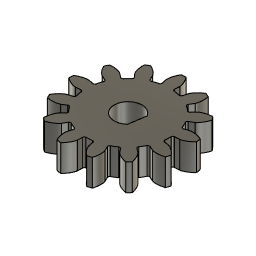
Spur Gear (13 teeth) (Autodesk Fusion 360 design; units mm, degrees)
description: Spur Gear; Module: 1.5; Num Teeth: 13; Pressure Angle: 20.0; Backlash: 0.15 mm
Autodesk Fusion 360 part; units mm, degrees
sketch "Sketch1" plane through (0, 0, 0) normal (0, 0, 1) x (1, 0, 0)
  circle A0 centre (0, 0) radius 7.8992
extrude "Extrude1" add sketch "Sketch1" along normal blind 5
sketch "Sketch2" plane through (0, 0, 0) normal (0, 0, 1) x (1, 0, 0)
  spline S0 degree 5 poles (9.0824, -1.2049) (9.0885, -1.2057) (9.1008, -1.2071) (9.1191, -1.2087) (9.1437, -1.2097) (9.1746, -1.2095) (9.2055, -1.2083) (9.2365, -1.2064) (9.2675, -1.2041) (9.2986, -1.2016) (9.3296, -1.1988) (9.3607, -1.1957) (9.3919, -1.1921) (9.423, -1.1881) (9.4542, -1.1835) (9.4854, -1.1784) (9.5166, -1.1729) (9.5478, -1.167) (9.5791, -1.1608) (9.6103, -1.1544) (9.6416, -1.1476) (9.6728, -1.1405) (9.7041, -1.1331) (9.7353, -1.1254) (9.7665, -1.1174) (9.7978, -1.109) (9.829, -1.1003) (9.8603, -1.0913) (9.8915, -1.0821) (9.9227, -1.0726) (9.9539, -1.0628) (9.9851, -1.0527) (10.0163, -1.0424) (10.0475, -1.0317) (10.0786, -1.0209) (10.1098, -1.0097) (10.1409, -0.9983) (10.172, -0.9866) (10.2031, -0.9747) (10.2342, -0.9626) (10.2652, -0.9501) (10.2962, -0.9375) (10.3272, -0.9246) (10.3582, -0.9114) (10.3892, -0.898) (10.4201, -0.8844) (10.451, -0.8706) (10.4819, -0.8565) (10.5127, -0.8421) (10.5435, -0.8276) (10.5743, -0.8128) (10.605, -0.7978) (10.6357, -0.7825) (10.6664, -0.7671) (10.6971, -0.7514) (10.7277, -0.7355) (10.7582, -0.7193) (10.7888, -0.703) (10.8193, -0.6864) (10.8497, -0.6696) (10.8801, -0.6526) (10.9105, -0.6354) (10.9409, -0.618) (10.9711, -0.6004) (11.0014, -0.5825) (11.0316, -0.5645) (11.0618, -0.5462) (11.0919, -0.5277) (11.1219, -0.5091) (11.1519, -0.4902) (11.1819, -0.4711) (11.2058, -0.4557) (11.2238, -0.444) (11.2357, -0.4362) (11.2417, -0.4323) knots 0 0 0 0 0 0 0.01428571 0.02857143 0.04285714 0.05714286 0.07142857 0.08571429 0.1 0.11428571 0.12857143 0.14285714 0.15714286 0.17142857 0.18571429 0.2 0.21428571 0.22857143 0.24285714 0.25714286 0.27142857 0.28571429 0.3 0.31428571 0.32857143 0.34285714 0.35714286 0.37142857 0.38571429 0.4 0.41428571 0.42857143 0.44285714 0.45714286 0.47142857 0.48571429 0.5 0.51428571 0.52857143 0.54285714 0.55714286 0.57142857 0.58571429 0.6 0.61428571 0.62857143 0.64285714 0.65714286 0.67142857 0.68571429 0.7 0.71428571 0.72857143 0.74285714 0.75714286 0.77142857 0.78571429 0.8 0.81428571 0.82857143 0.84285714 0.85714286 0.87142857 0.88571429 0.9 0.91428571 0.92857143 0.94285714 0.95714286 0.97142857 0.98571429 1 1 1 1 1 1
  spline S1 degree 5 poles (9.0824, 1.2049) (9.0885, 1.2057) (9.1008, 1.2071) (9.1191, 1.2087) (9.1437, 1.2097) (9.1746, 1.2095) (9.2055, 1.2083) (9.2365, 1.2064) (9.2675, 1.2041) (9.2986, 1.2016) (9.3296, 1.1988) (9.3607, 1.1957) (9.3919, 1.1921) (9.423, 1.1881) (9.4542, 1.1835) (9.4854, 1.1784) (9.5166, 1.1729) (9.5478, 1.167) (9.5791, 1.1608) (9.6103, 1.1544) (9.6416, 1.1476) (9.6728, 1.1405) (9.7041, 1.1331) (9.7353, 1.1254) (9.7665, 1.1174) (9.7978, 1.109) (9.829, 1.1003) (9.8603, 1.0913) (9.8915, 1.0821) (9.9227, 1.0726) (9.9539, 1.0628) (9.9851, 1.0527) (10.0163, 1.0424) (10.0475, 1.0317) (10.0786, 1.0209) (10.1098, 1.0097) (10.1409, 0.9983) (10.172, 0.9866) (10.2031, 0.9747) (10.2342, 0.9626) (10.2652, 0.9501) (10.2962, 0.9375) (10.3272, 0.9246) (10.3582, 0.9114) (10.3892, 0.898) (10.4201, 0.8844) (10.451, 0.8706) (10.4819, 0.8565) (10.5127, 0.8421) (10.5435, 0.8276) (10.5743, 0.8128) (10.605, 0.7978) (10.6357, 0.7825) (10.6664, 0.7671) (10.6971, 0.7514) (10.7277, 0.7355) (10.7582, 0.7193) (10.7888, 0.703) (10.8193, 0.6864) (10.8497, 0.6696) (10.8801, 0.6526) (10.9105, 0.6354) (10.9409, 0.618) (10.9711, 0.6004) (11.0014, 0.5825) (11.0316, 0.5645) (11.0618, 0.5462) (11.0919, 0.5277) (11.1219, 0.5091) (11.1519, 0.4902) (11.1819, 0.4711) (11.2058, 0.4557) (11.2238, 0.444) (11.2357, 0.4362) (11.2417, 0.4323) knots 0 0 0 0 0 0 0.01428571 0.02857143 0.04285714 0.05714286 0.07142857 0.08571429 0.1 0.11428571 0.12857143 0.14285714 0.15714286 0.17142857 0.18571429 0.2 0.21428571 0.22857143 0.24285714 0.25714286 0.27142857 0.28571429 0.3 0.31428571 0.32857143 0.34285714 0.35714286 0.37142857 0.38571429 0.4 0.41428571 0.42857143 0.44285714 0.45714286 0.47142857 0.48571429 0.5 0.51428571 0.52857143 0.54285714 0.55714286 0.57142857 0.58571429 0.6 0.61428571 0.62857143 0.64285714 0.65714286 0.67142857 0.68571429 0.7 0.71428571 0.72857143 0.74285714 0.75714286 0.77142857 0.78571429 0.8 0.81428571 0.82857143 0.84285714 0.85714286 0.87142857 0.88571429 0.9 0.91428571 0.92857143 0.94285714 0.95714286 0.97142857 0.98571429 1 1 1 1 1 1
  arc A0 (11.2417, -0.4323) -> (11.2417, 0.4323) centre (0, 0) ccw
  line L0 (7.8207, -1.0388) -> (9.0824, -1.2049)
  line L1 (7.8207, 1.0388) -> (9.0824, 1.2049)
  line L2 (7.8207, -1.0388) -> (7.8207, 1.0388)
  point P0 (9.2326, -1.2065)
  point P1 (9.3848, -1.1929)
  point P2 (9.5381, -1.1688)
  point P3 (9.6922, -1.1359)
  point P4 (9.847, -1.0951)
  point P5 (10.0022, -1.047)
  point P6 (10.1577, -0.992)
  point P7 (10.3133, -0.9304)
  point P8 (10.4688, -0.8624)
  point P9 (10.6242, -0.7882)
  point P10 (10.7793, -0.708)
  point P11 (10.934, -0.6219)
  point P12 (11.0882, -0.5299)
  point P13 (9.2326, 1.2065)
  point P14 (9.3848, 1.1929)
  point P15 (9.5381, 1.1688)
  point P16 (9.6922, 1.1359)
  point P17 (9.847, 1.0951)
  point P18 (10.0022, 1.047)
  point P19 (10.1577, 0.992)
  point P20 (10.3133, 0.9304)
  point P21 (10.4688, 0.8624)
  point P22 (10.6242, 0.7882)
  point P23 (10.7793, 0.708)
  point P24 (10.934, 0.6219)
  point P25 (11.0882, 0.5299)
extrude "Extrude2" add sketch "Sketch2" along normal blind 5
fillet "Fillet1" radius 0.303 2 edges at (7.8304, -1.0401, 2.5) (7.8304, 1.0401, 2.5)
pattern_circular "C-Pattern1" count 13 over 360 about axis through (0, 0, 0) along (0, 0, 1) of "Extrude2", "Fillet1"
sketch "Sketch3" plane through (0, 0, 0) normal (0, 0, 1) x (1, 0, 0)
  circle A0 centre (0, 0) radius 9.75 construction
move_body "Move1" bodies 1 to x (1, 0, 0) y (0, 1, 0) z (0, 0, 1) at (33.5494, 0, 2.5)
move_body "Move2" bodies 1 to x (0.939693, 0.34202, 0) y (-0.34202, 0.939693, 0) z (0, 0, 1) at (2.0233, -11.4746, 0)
sketch "sketch 709" plane through (0, 0, 7.5) normal (0, 0, 1) x (-1, 0, 0)
  arc A0 (-35.5994, -1.5992) -> (-35.5994, 1.5992) centre (-33.5494, 0) ccw
  line L0 (-35.5994, -1.5992) -> (-35.5994, 1.5992)
extrude "Extrude3" cut sketch "sketch 709" against normal blind 5
move_body "Move3" bodies 1 to x (0.987688, -0.156434, 0) y (0.156434, 0.987688, 0) z (0, 0, 1) at (0.413, 5.2483, 0)
